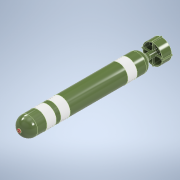
# Autodesk Inventor part: torpedo
Saved by Autodesk Inventor 2022 (Build 260153000, 153)
## iProperties
Created: 2021-12-16
Part Number: torpedo
Material: Generic
Document SubType Name: Modeling
Designer: jpc
Density: 1 g/cm^3
Appearance: Dark Olive
Author: jpc
Autodesk Inventor part; units mm, degrees
ref_plane "YZ Plane" through (0, 0, 0) normal (1, 0, 0) x (0, 1, 0)
ref_plane "XZ Plane" through (0, 0, 0) normal (0, 1, 0) x (-1, 0, 0)
sketch "Sketch1" plane through (0, 0, 0) normal (1, 0, 0) x (0, 1, 0)
  arc A0 (0, 625) -> (40, 631.5728) centre (0, 750) ccw
  line L0 (125, 750) -> (40, 750) construction
  line L1 (0, 750) -> (0, 625)
  line L2 (0, -750) -> (40, -750)
  line L3 (125, -750) -> (125, 750)
  line L4 (0, -750) -> (40, -750)
  line L5 (40, -750) -> (40, -835) construction
  line L6 (40, -1050) -> (0, -1050)
  line L7 (0, -1050) -> (0, -750)
  line L8 (125, -750) -> (40, -835)
  arc A1 (125, 750) -> (0, 875) centre (0, 750) ccw
  arc A2 (0, 875) -> (0, 625) centre (0, 750) ccw construction
  arc A3 (40, 631.5728) -> (125, 750) centre (0, 750) ccw construction
  line L9 (0, 625) -> (0, -750)
  line L10 (40, 750) -> (0, 750)
  line L11 (40, -750) -> (125, -750) construction
  line L12 (40, -835) -> (40, -1050)
  line L13 (0, 875) -> (0, 750)
  line L14 (125, 0) -> (0, 0)
  dimension "d1" = 1500
  dimension "d2" = 300
  dimension "d3" = 40
  dimension "d4" = 45
  dimension "d6" = 250
  constraints: 30 end point, 9 parallel, 8 point on circle, 7 perpendicular, 4 centre point, 4 point on line, 3 horizontal, 2 coincident, 1 collinear, 1 midpoint
  measures "d1" distance of L3.start L0.start
  measures "d2" distance of L2.end L6.start
  measures "d3" distance of L6.start L6.end
  measures "d4" angle of L5 L8
  measures "d6" diameter of L3 L9
revolve "Revolution1" add sketch "Sketch1" angle 360 about axis through (0, 0, 625) along (0, 0, -1)
fillet "Fillet1" radius 75 2 edges at (0, -125, -750) (0, -40, -835)
sketch "Sketch2" plane through (0, 0, 0) normal (0, 1, 0) x (-1, 0, 0)
  line L0 (-135, -927.3773) -> (-125, -927.3773)
  line L1 (-125, -927.3773) -> (-125, -1050)
  line L2 (-125, -1050) -> (-135, -1050)
  line L3 (-135, -1050) -> (-135, -927.3773)
  line L4 (-40, -1050) -> (40, -1050) projected
  line L5 (40, -866.066) -> (-40, -866.066) construction
  line L6 (-125, 750) -> (125, 750) projected
  line L7 (-125, -718.934) -> (125, -718.934) construction
  line L8 (0, -866.066) -> (0, -1050)
  point P0 (0, 0)
  dimension "d8" = 183.934
  dimension "d9" = 122.6227
  dimension "d10" = 250
  dimension "d11" = 250
  dimension "d12" = 80
  dimension "d13" = 10
  constraints: 10 end point, 2 midpoint, 2 parallel, 1 collinear, 1 horizontal, 1 perpendicular
  measures "d8" distance between parallel lines of L4 L5
  measures "d9" distance of L2.end L0.start
  measures "d10" distance of L7.start L7.end
  measures "d11" diameter of L1 L8
  measures "d12" distance of L4.start L4.end
  measures "d13" distance of L1.end L2.end
revolve "Revolution2" add sketch "Sketch2" angle 360 about axis through (0, 0, -866.066) along (0, 0, -1)
sketch "Sketch3" plane through (0, 0, -1050) normal (0, 0, -1) x (-1, 0, 0)
  line L0 (148.5, 5) -> (-148.5, 5)
  line L1 (-148.5, 5) -> (-148.5, -5)
  line L2 (-148.5, -5) -> (148.5, -5)
  line L3 (148.5, -5) -> (148.5, 5)
  line L4 (148.5, 5) -> (-148.5, -5) construction
  circle A0 centre (0, 0) radius 135 construction
  circle A1 centre (0, 0) radius 125 construction
  line L5 (5, 148.5) -> (-5, 148.5)
  line L6 (-5, 148.5) -> (-5, -148.5)
  line L7 (-5, -148.5) -> (5, -148.5)
  line L8 (5, -148.5) -> (5, 148.5)
  line L9 (5, 148.5) -> (-5, -148.5) construction
  point P0 (0, 0)
  point P1 (0, 0)
  point P2 (5, -5)
  point P3 (5, 5)
  point P4 (-5, 5)
  point P5 (-5, -5)
  dimension "d15" = 270
  dimension "d16" = 250
  dimension "d17" = 10
  dimension "d18" = 297
  dimension "d19" = 10
  dimension "d20" = 297
  constraints: 20 end point, 4 parallel, 2 horizontal, 2 midpoint, 2 perpendicular, 1 coincident
  measures "d15" diameter of A0
  measures "d16" diameter of A1
  measures "d17" distance of L2.end L0.start
  measures "d18" distance of L1.end L2.end
  measures "d19" distance of L6.end L7.end
  measures "d20" distance of L5.end L6.end
extrude "Extrusion1" add sketch "Sketch3" against normal up to surface (122.6227 mm away)
sketch "Sketch4" plane through (0, 0, 0) normal (1, 0, 0) x (0, 1, 0)
  line L0 (148.5, -927.3773) -> (148.5, -1050) construction
  line L1 (148.5, -1050) -> (-148.5, -1050) construction
  line L2 (-148.5, -1050) -> (-148.5, -927.3773) construction
  line L3 (-148.5, -927.3773) -> (-40, -927.3773) construction
  line L4 (-40, -927.3773) -> (-40, -866.066) construction
  arc A0 (-40, -866.066) -> (-61.967, -813.033) centre (-115, -866.066) ccw construction
  line L5 (-61.967, -813.033) -> (-103.033, -771.967) construction
  arc A1 (-125, -718.934) -> (-103.033, -771.967) centre (-50, -718.934) ccw construction
  line L6 (-125, -718.934) -> (-125, 750) construction
  arc A2 (0, 875) -> (-125, 750) centre (0, 750) ccw construction
  arc A3 (125, 750) -> (0, 875) centre (0, 750) ccw construction
  line L7 (125, 750) -> (125, -718.934) construction
  arc A4 (103.033, -771.967) -> (125, -718.934) centre (50, -718.934) ccw construction
  line L8 (103.033, -771.967) -> (61.967, -813.033) construction
  arc A5 (61.967, -813.033) -> (40, -866.066) centre (115, -866.066) ccw construction
  line L9 (40, -866.066) -> (40, -927.3773) construction
  line L10 (40, -927.3773) -> (148.5, -927.3773) construction
  line L11 (39.6863, -927.3773) -> (39.6863, -1050) construction
  line L12 (39.6863, -927.3773) -> (124.9, -927.3773) construction
  line L13 (124.9, -1050) -> (124.9, -927.3773) construction
  line L14 (39.6863, -1050) -> (124.9, -1050) construction
  line L15 (124.9, -1050) -> (124.9, -927.3773) projected
  line L16 (124.9, -950.9774) -> (39.6863, -950.9774)
  line L17 (39.6863, -950.9774) -> (39.6863, -1026.4) construction
  line L18 (39.6863, -1026.4) -> (124.9, -1026.4)
  line L19 (124.9, -1026.4) -> (124.9, -950.9774)
  line L20 (0, -1440.1777) -> (0, 1291.066) projected
  line L21 (39.6863, -950.9774) -> (23.6, -950.9774)
  line L22 (23.6, -950.9774) -> (23.6, -1026.4)
  line L23 (23.6, -1026.4) -> (39.6863, -1026.4)
  line L24 (39.6863, -1026.4) -> (39.6863, -950.9774) construction
  point P0 (0, 0)
  dimension "d23" = 23.6
  dimension "d24" = 23.6
  dimension "d25" = 23.6
  dimension "d27" = 23.6
  constraints: 16 end point, 4 parallel, 2 horizontal, 2 perpendicular, 2 point on line
  measures "d23" distance between parallel lines of L13 L0
  measures "d24" distance between parallel lines of L12 L16
  measures "d25" distance between parallel lines of L1 L18
  measures "d27" distance between parallel lines of L22 L20
revolve "Revolution3" cut sketch "Sketch4" angle 360 about axis through (0, 0, -10) along (0, 0, 1)
sketch "Sketch5" plane through (0, 0, 0) normal (1, 0, 0) x (0, 1, 0)
  line L0 (-124.9, -1026.4) -> (-23.6, -1026.4) construction
  line L1 (-23.6, -1026.4) -> (-23.6, -950.9774) construction
  line L2 (-23.6, -950.9774) -> (-124.9, -950.9774) construction
  line L3 (-124.9, -950.9774) -> (-124.9, -1026.4) construction
  line L4 (23.6, -1026.4) -> (124.9, -1026.4) construction
  line L5 (124.9, -1026.4) -> (124.9, -950.9774) construction
  line L6 (124.9, -950.9774) -> (23.6, -950.9774) construction
  line L7 (23.6, -950.9774) -> (23.6, -1026.4) construction
  line L8 (148.5, -927.3773) -> (148.5, -1050) construction
  line L9 (148.5, -1050) -> (-148.5, -1050) construction
  line L10 (-148.5, -1050) -> (-148.5, -927.3773) construction
  line L11 (-148.5, -927.3773) -> (-40, -927.3773) construction
  line L12 (-40, -927.3773) -> (-40, -866.066) construction
  arc A0 (-40, -866.066) -> (-61.967, -813.033) centre (-115, -866.066) ccw construction
  line L13 (-61.967, -813.033) -> (-103.033, -771.967) construction
  arc A1 (-125, -718.934) -> (-103.033, -771.967) centre (-50, -718.934) ccw construction
  line L14 (-125, -718.934) -> (-125, 750) construction
  arc A2 (0, 875) -> (-125, 750) centre (0, 750) ccw construction
  arc A3 (125, 750) -> (0, 875) centre (0, 750) ccw construction
  line L15 (125, 750) -> (125, -718.934) construction
  arc A4 (103.033, -771.967) -> (125, -718.934) centre (50, -718.934) ccw construction
  line L16 (103.033, -771.967) -> (61.967, -813.033) construction
  arc A5 (61.967, -813.033) -> (40, -866.066) centre (115, -866.066) ccw construction
  line L17 (40, -866.066) -> (40, -927.3773) construction
  line L18 (40, -927.3773) -> (148.5, -927.3773) construction
  line L19 (0, 750) -> (25, 750)
  line L20 (25, 750) -> (25, 887.5)
  line L21 (25, 887.5) -> (0, 887.5)
  line L22 (0, 887.5) -> (0, 750)
  point P0 (0, 0)
  dimension "d28" = 125
  dimension "d29" = 137.5
  dimension "d30" = 25
  constraints: 8 end point, 2 parallel, 1 horizontal, 1 perpendicular
  measures "d28" radius of A3
  measures "d29" distance of L19.end L20.end
  measures "d30" distance of L20.end L21.end
revolve "Revolution4" add sketch "Sketch5" angle 360 about axis through (0, 0, 887.5) along (0, 0, -1)
fillet "Face Fillet1" radius 10 1 edges at (0, -25, 887.5)
sketch "Sketch6" plane through (0, 0, 0) normal (1, 0, 0) x (0, 1, 0)
  line L0 (-124.9, -1026.4) -> (-23.6, -1026.4) construction
  line L1 (-23.6, -1026.4) -> (-23.6, -950.9774) construction
  line L2 (-23.6, -950.9774) -> (-124.9, -950.9774) construction
  line L3 (-124.9, -950.9774) -> (-124.9, -1026.4) construction
  line L4 (23.6, -1026.4) -> (124.9, -1026.4) construction
  line L5 (124.9, -1026.4) -> (124.9, -950.9774) construction
  line L6 (124.9, -950.9774) -> (23.6, -950.9774) construction
  line L7 (23.6, -950.9774) -> (23.6, -1026.4) construction
  line L8 (148.5, -927.3773) -> (148.5, -1050) projected
  line L9 (148.5, -1050) -> (-148.5, -1050) construction
  line L10 (-148.5, -1050) -> (-148.5, -927.3773) construction
  line L11 (-148.5, -927.3773) -> (-40, -927.3773) construction
  line L12 (-40, -927.3773) -> (-40, -866.066) construction
  arc A0 (-40, -866.066) -> (-61.967, -813.033) centre (-115, -866.066) ccw construction
  line L13 (-61.967, -813.033) -> (-103.033, -771.967) construction
  arc A1 (-125, -718.934) -> (-103.033, -771.967) centre (-50, -718.934) ccw construction
  line L14 (-125, -718.934) -> (-125, 750) construction
  arc A2 (-25, 872.4745) -> (-125, 750) centre (0, 750) ccw construction
  line L15 (-25, 872.4745) -> (-25, 877.5) construction
  arc A3 (-15, 887.5) -> (-25, 877.5) centre (-15, 877.5) ccw construction
  line L16 (-15, 887.5) -> (15, 887.5) construction
  arc A4 (25, 877.5) -> (15, 887.5) centre (15, 877.5) ccw construction
  line L17 (25, 877.5) -> (25, 872.4745) construction
  arc A5 (125, 750) -> (25, 872.4745) centre (0, 750) ccw construction
  line L18 (125, 750) -> (125, -718.934) construction
  arc A6 (103.033, -771.967) -> (125, -718.934) centre (50, -718.934) ccw construction
  line L19 (103.033, -771.967) -> (61.967, -813.033) construction
  arc A7 (61.967, -813.033) -> (40, -866.066) centre (115, -866.066) ccw construction
  line L20 (40, -866.066) -> (40, -927.3773) construction
  line L21 (40, -927.3773) -> (148.5, -927.3773) construction
  line L22 (125, 750) -> (125, -718.934) construction
  line L23 (125, 625) -> (126.25, 625)
  line L24 (126.25, 625) -> (126.25, 500)
  line L25 (126.25, 500) -> (125, 500)
  line L26 (125, 500) -> (125, 625)
  line L27 (125, 437.5) -> (126.25, 437.5)
  line L28 (126.25, 437.5) -> (126.25, 312.5)
  line L29 (126.25, 312.5) -> (125, 312.5)
  line L30 (125, 312.5) -> (125, 437.5)
  line L31 (125, -468.934) -> (126.25, -468.934)
  line L32 (126.25, -468.934) -> (126.25, -593.934)
  line L33 (126.25, -593.934) -> (125, -593.934)
  line L34 (125, -593.934) -> (125, -468.934)
  line L35 (0, -1438.0588) -> (0, 1278.353) projected
  point P0 (0, 0)
  dimension "d33" = 125
  dimension "d34" = 125
  dimension "d35" = 125
  dimension "d36" = 125
  dimension "d37" = 125
  dimension "d38" = 125
  dimension "d39" = 62.5
  dimension "d40" = 1.25
  constraints: 24 end point, 6 parallel, 5 point on line, 3 horizontal, 3 perpendicular
  measures "d33" radius of A5
  measures "d34" distance of L23.end L24.end
  measures "d35" distance of L27.end L28.end
  measures "d36" distance of L31.end L32.end
  measures "d37" distance from line of L33 A6.centre
  measures "d38" horizontal distance of L23.start A2.centre
  measures "d39" vertical distance of L27.end L25.end
  measures "d40" distance between parallel lines of L26 L24
revolve "Revolution5" add sketch "Sketch6" angle 360 about axis through (0, 0, -10) along (0, 0, 1) separate body
ref_plane "Work Plane2" through (-124.7998, 5, -988.6887) normal (0, 0, 1) x (1, 0, 0)
sketch "Sketch7" plane through (-124.7998, 5, -988.6887) normal (0, 0, 1) x (1, 0, 0)
  line L0 (136.6557, 10.1736) -> (165.8771, 60.4775) construction
  line L1 (165.8771, 60.4775) -> (149.3262, 85.1315) construction
  line L2 (149.3262, 85.1315) -> (157.6016, 108.4772) construction
  line L3 (157.6016, 108.4772) -> (200.9938, 101.9347) construction
  line L4 (200.9938, 101.9347) -> (234.4744, 60.4775) construction
  line L5 (234.4744, 60.4775) -> (135.4834, 2.3861) construction
  spline S0 degree 4 poles (136.6557, 10.1736) (165.8771, 60.4775) (149.3262, 85.1315) (157.6016, 108.4772) (200.9938, 101.9347) (234.4744, 60.4775) (135.4834, 2.3861) knots 1 1 1 1 1 2 3 4 4 4 4 4
  line L6 (135.4834, 2.3861) -> (136.6557, 10.1736)
  point P0 (124.7998, -5)
  constraints: 2 end point, 3 other
extrude "Extrusion2" add sketch "Sketch7" along normal mid plane 10 bodies 1
fillet "Fillet2" radius 2.5 2 edges at (42.4422, 104.9993, -983.6887) (42.4422, 104.9993, -993.6887)
pattern_circular "Circular Pattern2" count 4 over 360 about axis through (0, 0, -10) along (0, 0, 1) of "Extrusion2", "Fillet2" bodies 1
equation "\"d2\" = 0.2 * d1"
equation "\"d3\" = 0.08 * d0"
equation "\"d9\" = 0.666667 * d8"
equation "\"d11\" = d10"
equation "\"d13\" = 0.125 * d12"
equation "\"d17\" = -0.5 * d16 + 0.5 * d15"
equation "\"d18\" = 1.1 * d15"
equation "\"d19\" = d17"
equation "\"d20\" = d18"
equation "\"d24\" = d23"
equation "\"d25\" = d24"
equation "\"d27\" = d25"
equation "\"d29\" = 1.1 * d28"
equation "\"d30\" = 0.2 * d28"
equation "\"d34\" = d33"
equation "\"d35\" = d34"
equation "\"d36\" = d35"
equation "\"d37\" = d36"
equation "\"d38\" = d34"
equation "\"d39\" = 0.5 * d38"
equation "\"d40\" = 0.01 * d33"
equation "\"d0\" = 500"
body "Solid1"
body "Solid2"
